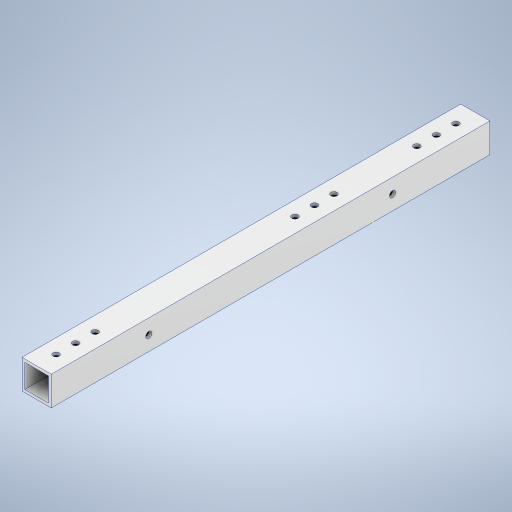
# Autodesk Inventor part: 射出_角柱3
Saved by Autodesk Inventor 2023 (Build 270158000, 158)
## iProperties
Created: 2022-04-20
Part Number: 射出_角柱3
Material: アルミニウム 6061
Document SubType Name: Modeling
Designer: yuta
Density: 2.7 g/cm^3
Appearance: アルミニウム - フラット
Mass: 48.6212 g
Surface Area: 244.439 cm^2
Volume: 18.0079 cm^3
Author: yuta
Autodesk Inventor part; units mm, degrees
ref_plane "YZ Plane" through (0, 0, 0) normal (1, 0, 0) x (0, 1, 0)
ref_plane "XZ Plane" through (0, 0, 0) normal (0, 1, 0) x (-1, 0, 0)
ref_plane "XY Plane" through (0, 0, 0) normal (0, 0, 1) x (1, 0, 0)
sketch "スケッチ1" plane through (0, 0, 0) normal (0, 0, 1) x (1, 0, 0)
  line L0 (0, 0) -> (15, 0)
  line L1 (15, 0) -> (15, 15)
  line L2 (15, 15) -> (0, 15)
  line L3 (0, 15) -> (0, 0)
  dimension "d0" = 15
  dimension "d1" = 15
  constraints: 8 end point, 2 parallel, 1 horizontal, 1 perpendicular
  measures "d0" distance of L2.end L1.end
  measures "d1" distance of L1.end L0.end
extrude "押し出し1" add sketch "スケッチ1" along normal blind 150
sketch "スケッチ2" plane through (0, 0, 0) normal (0, 0, -1) x (-1, 0, 0)
  line L0 (0, 0) -> (-15, 0)
  line L1 (-15, 0) -> (-15, 15)
  line L2 (-15, 15) -> (0, 15)
  line L3 (0, 15) -> (0, 0)
  dimension "d4" = 15
  dimension "d5" = 15
  constraints: 8 end point, 2 parallel, 1 horizontal, 1 perpendicular
  measures "d4" distance of L1.end L2.end
  measures "d5" distance of L0.end L1.end
extrude "押し出し2" cut sketch "スケッチ2" against normal blind 30
sketch "スケッチ4" plane through (0, 0, 30) normal (0, 0, -1) x (-1, 0, 0)
  line L0 (0, 0) -> (-15, 0) projected
  line L1 (-15, 15) -> (0, 15) projected
  line L2 (0, 0) -> (-15, 0)
  line L3 (-15, 0) -> (-15, 15)
  line L4 (-15, 15) -> (0, 15)
  line L5 (0, 15) -> (0, 0)
  dimension "d8" = 15
  dimension "d9" = 15
  constraints: 8 end point, 2 parallel, 1 horizontal, 1 perpendicular
  measures "d8" distance of L1.start L4.end
  measures "d9" distance of L2.end L1.start
extrude "押し出し3" add sketch "スケッチ4" along normal blind 15
sketch "スケッチ5" plane through (0, 0, 150) normal (0, 0, 1) x (1, 0, 0)
  line L0 (0, 0) -> (15, 0)
  line L1 (15, 0) -> (15, 15)
  line L2 (15, 15) -> (0, 15)
  line L3 (0, 15) -> (0, 0)
  dimension "d14" = 15
  dimension "d15" = 15
  constraints: 8 end point, 2 parallel, 1 horizontal, 1 perpendicular
  measures "d14" distance of L2.end L1.end
  measures "d15" distance of L1.end L0.end
extrude "押し出し4" add sketch "スケッチ5" along normal blind 15
sketch "スケッチ6" plane through (0, 0, 15) normal (0, 0, -1) x (-1, 0, 0)
  line L0 (-15, 0) -> (0, 0) projected
  line L1 (0, 0) -> (-15, 0)
  line L2 (-15, 0) -> (-15, 15)
  line L3 (-15, 15) -> (0, 15)
  line L4 (0, 15) -> (0, 0)
  dimension "d18" = 15
  dimension "d19" = 15
  constraints: 8 end point, 2 parallel, 1 horizontal, 1 perpendicular
  measures "d18" distance of L2.end L3.end
  measures "d19" distance of L1.end L2.end
extrude "押し出し5" add sketch "スケッチ6" along normal blind 55
sketch "スケッチ7" plane through (0, 0, -40) normal (0, 0, -1) x (-1, 0, 0)
  line L0 (0, 0) -> (-15, 0)
  line L1 (-15, 0) -> (-15, 15)
  line L2 (-15, 15) -> (0, 15)
  line L3 (0, 15) -> (0, 0)
  dimension "d22" = 15
  dimension "d23" = 15
  constraints: 8 end point, 2 parallel, 1 horizontal, 1 perpendicular
  measures "d22" distance of L1.end L2.end
  measures "d23" distance of L0.end L1.end
extrude "押し出し6" add sketch "スケッチ7" along normal blind 3
sketch "スケッチ8" plane through (0, 0, -43) normal (0, 0, -1) x (-1, 0, 0)
  line L0 (0, 0) -> (-15, 0)
  line L1 (-15, 0) -> (-15, 15)
  line L2 (-15, 15) -> (0, 15)
  line L3 (0, 15) -> (0, 0)
  dimension "d26" = 15
  dimension "d27" = 15
  constraints: 8 end point, 2 parallel, 1 horizontal, 1 perpendicular
  measures "d26" distance of L1.end L2.end
  measures "d27" distance of L0.end L1.end
extrude "押し出し7" add sketch "スケッチ8" along normal blind 2
sketch "スケッチ9" plane through (0, 15, 165) normal (0, 1, 0) x (1, 0, 0)
  circle A0 centre (7.5, 142.5) radius 1.6
  line L0 (0, 210) -> (15, 210) projected
  line L1 (0, 210) -> (0, 0) projected
  point P0 (0, 165)
  dimension "d30" = 3.2
  dimension "d31" = 67.5
  dimension "d32" = 7.5
  constraints: 1 centre point
  measures "d30" diameter of A0
  measures "d31" distance from line of L0 A0.centre
  measures "d32" distance from line of L1 A0.centre
hole "穴1" at (7.5, 15, 22.5) direction (0, -1, 0) diameter 3.2 end through all
sketch "スケッチ10" plane through (0, 0, -45) normal (0, 0, -1) x (-1, 0, 0)
  line L0 (0, 0) -> (-15, 0)
  line L1 (-15, 0) -> (-15, 15)
  line L2 (-15, 15) -> (0, 15)
  line L3 (0, 15) -> (0, 0)
  constraints: 8 end point, 2 parallel, 1 horizontal, 1 perpendicular
extrude "押し出し8" add sketch "スケッチ10" along normal blind 15
sketch "スケッチ11" plane through (0, 15, 165) normal (0, 1, 0) x (1, 0, 0)
  line L0 (0, 225) -> (15, 225) projected
  line L1 (0, 225) -> (0, 0) projected
  point P0 (0, 165)
  point P1 (7.5, 215)
  point P2 (7.5, 205)
  point P3 (7.5, 195)
  dimension "d42" = 10
  dimension "d43" = 7.5
  dimension "d44" = 10
  dimension "d45" = 10
  measures "d42" distance from line of L0 point (7.5, 215)
  measures "d43" distance from line of L1 point (7.5, 215)
  measures "d44" distance of point (7.5, 215) point (7.5, 205)
  measures "d45" distance of point (7.5, 205) point (7.5, 195)
hole "穴2" at (7.5, 15, -50) at (7.5, 15, -40) at (7.5, 15, -30) direction (0, -1, 0) diameter 3.2 end through all
sketch "スケッチ12" plane through (15, 0, 165) normal (1, 0, 0) x (0, 0, -1)
  point P0 (165, 0)
sketch "スケッチ13" plane through (0, 15, 165) normal (0, 1, 0) x (1, 0, 0)
  line L0 (0, 225) -> (0, 0) projected
  line L1 (15, 0) -> (0, 0) projected
  line L2 (15, 225) -> (15, 0) projected
  point P0 (0, 165)
  point P1 (7.5, 10)
  point P2 (7.5, 20)
  point P3 (7.5, 30)
  dimension "d53" = 7.5
  dimension "d54" = 10
  dimension "d55" = 10
  dimension "d56" = 10
  dimension "d57" = 7.5
  dimension "d58" = 7.5
  measures "d53" distance from line of L0 point (7.5, 10)
  measures "d54" distance from line of L1 point (7.5, 10)
  measures "d55" distance of point (7.5, 10) point (7.5, 20)
  measures "d56" distance of point (7.5, 20) point (7.5, 30)
  measures "d57" distance from line of L2 point (7.5, 20)
  measures "d58" distance from line of L2 point (7.5, 30)
hole "穴3" at (7.5, 15, 155) at (7.5, 15, 145) at (7.5, 15, 135) direction (0, -1, 0) diameter 3.2 end through all
sketch "スケッチ14" plane through (0, 15, 165) normal (0, 1, 0) x (1, 0, 0)
  circle A0 centre (7.5, 142.5) radius 1.6 projected
  line L0 (0, 225) -> (0, 0) projected
  line L1 (15, 225) -> (15, 0) projected
  point P0 (0, 165)
  point P1 (7.5, 152.5)
  point P2 (7.5, 132.5)
  dimension "d66" = 10
  dimension "d67" = 7.5
  dimension "d68" = 10
  dimension "d69" = 7.5
  measures "d66" distance of A0.centre point (7.5, 152.5)
  measures "d67" distance from line of L0 point (7.5, 152.5)
  measures "d68" distance of point (7.5, 132.5) A0.centre
  measures "d69" distance from line of L1 point (7.5, 132.5)
hole "穴4" at (7.5, 15, 32.5) at (7.5, 15, 12.5) direction (0, -1, 0) diameter 3.2 end through all
sketch "スケッチ15" plane through (0, 0, 165) normal (0, 0, 1) x (1, 0, 0)
  line L0 (1.5, 1.5) -> (13.5, 1.5)
  line L1 (13.5, 1.5) -> (13.5, 13.5)
  line L2 (13.5, 13.5) -> (1.5, 13.5)
  line L3 (1.5, 13.5) -> (1.5, 1.5)
  line L4 (0, 0) -> (15, 0) projected
  line L5 (0, 15) -> (0, 0) projected
  dimension "d77" = 12
  dimension "d78" = 12
  dimension "d79" = 1.5
  dimension "d80" = 1.5
  constraints: 8 end point, 2 parallel, 1 horizontal, 1 perpendicular
  measures "d77" distance of L2.end L1.end
  measures "d78" distance of L1.end L0.end
  measures "d79" distance between parallel lines of L4 L0
  measures "d80" distance between parallel lines of L5 L3
extrude "押し出し9" cut sketch "スケッチ15" against normal blind 1400
sketch "スケッチ16" plane through (15, 0, 165) normal (1, 0, 0) x (0, 0, -1)
  line L0 (225, 15) -> (0, 15) projected
  line L1 (225, 15) -> (225, 0) projected
  line L2 (0, 0) -> (0, 15) projected
  line L3 (225, 0) -> (0, 0) projected
  point P0 (165, 0)
  point P1 (175, 7.5)
  point P2 (50, 7.5)
  point P3 (0, 7.5)
  dimension "d83" = 7.5
  dimension "d84" = 50
  dimension "d85" = 50
  dimension "d86" = 7.5
  constraints: 1 midpoint
  measures "d83" distance from line of point (175, 7.5) L0
  measures "d84" distance from line of L1 point (175, 7.5)
  measures "d85" distance of point (0, 7.5) point (50, 7.5)
  measures "d86" distance from line of L3 point (50, 7.5)
hole "穴5" at (15, 7.5, 115) at (15, 7.5, -10) direction (-1, 0, 0) diameter 3.2 end through all
